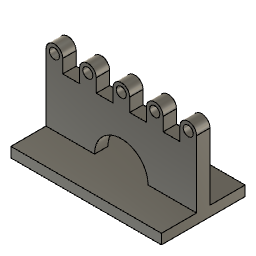
Model 3 (Autodesk Fusion 360 design; units mm, degrees)
Autodesk Fusion 360 part; units mm, degrees
note: some values were not read from the file. Set by a fixed rule: which sketch regions a step uses.
sketch "Sketch5" plane through (0, 0, 0) normal (0, 0, 1) x (1, 0, 0)
  line L0 (0, 0) -> (225, 0)
  line L1 (225, 0) -> (225, -125)
  line L2 (225, -125) -> (0, -125)
  line L3 (0, -125) -> (0, 0)
  dimension "d26" = 225
  dimension "d27" = 125
  constraint horizontal L0
  constraint vertical L1
  constraint horizontal L2
  constraint vertical L3
  constraint coincident L0.start L3.end
  measures "d26" distance of L0.start L0.end
  measures "d27" distance of L0.start L2.end
extrude "Extrude3" add sketch "Sketch5" along normal blind 15
sketch "Sketch6" plane through (0, 0, 15) normal (0, 0, 1) x (-1, 0, 0)
  line L0 (0, 125) -> (-225, 125)
  line L1 (-225, 125) -> (-225, 0)
  line L2 (-225, 0) -> (0, 0)
  line L3 (0, 0) -> (0, 125)
  line L4 (0, 0) -> (0, 62.5) construction
  line L5 (0, 62.5) -> (-225, 62.5) construction
  line L6 (0, 62.5) -> (0, 52.5)
  line L7 (0, 62.5) -> (0, 72.5)
  line L8 (0, 52.5) -> (-225, 52.5)
  line L9 (-225, 52.5) -> (-225, 72.5)
  line L10 (-225, 72.5) -> (0, 72.5)
  dimension "d30" = 62.5
  dimension "d31" = 10
  dimension "d32" = 10
  dimension "d33" = 225
  dimension "d34" = 20
  constraint coincident L2.end L3.start
  constraint perpendicular L0 L4
  constraint midpoint L1 L5.end
  constraint perpendicular L5 L6
  constraint perpendicular L5 L7
  constraint perpendicular L1 L8
  constraint perpendicular L5 L9
  measures "d30" distance of L2.end L4.end
  measures "d31" distance of L4.end L6.end
  measures "d32" distance of L4.end L7.end
  measures "d33" distance of L6.end L8.end
  measures "d34" distance of L8.end L9.end
extrude "Extrude4" add sketch "Sketch6" along normal blind 100 contours L1 L3 L6 L7 L8 L9 L10
sketch "Sketch7" plane through (0, -72.5, 0) normal (0, -1, 0) x (1, 0, 0)
  line L0 (0, 15) -> (225, 15)
  line L1 (225, 15) -> (225, 115)
  line L2 (225, 115) -> (0, 115)
  line L3 (0, 115) -> (0, 15)
  line L4 (0, 15) -> (72.5, 15) construction
  arc A0 (152.5, 15) -> (72.5, 15) centre (112.5, 15) ccw
  line L5 (0, 115) -> (25, 115)
  line L6 (25, 115) -> (50, 115)
  line L7 (50, 115) -> (75, 115)
  line L8 (75, 115) -> (100, 115)
  line L9 (100, 115) -> (125, 115)
  line L10 (125, 115) -> (150, 115)
  line L11 (150, 115) -> (175, 115)
  line L12 (175, 115) -> (200, 115)
  line L13 (200, 115) -> (225, 115)
  circle A1 centre (12.5, 115) radius 7.5
  circle A2 centre (62.5, 115) radius 7.5
  circle A3 centre (112.5, 115) radius 7.5
  circle A4 centre (162.5, 115) radius 7.5
  circle A5 centre (212.5, 115) radius 7.5
  line L14 (25, 115) -> (25, 95)
  line L15 (25, 95) -> (50, 95)
  line L16 (50, 95) -> (50, 115)
  line L17 (75, 115) -> (75, 95)
  line L18 (75, 95) -> (100, 95)
  line L19 (100, 95) -> (100, 115)
  line L20 (125, 115) -> (125, 95)
  line L21 (125, 95) -> (150, 95)
  line L22 (150, 95) -> (150, 115)
  line L23 (175, 115) -> (175, 95)
  line L24 (175, 95) -> (200, 95)
  line L25 (200, 95) -> (200, 115)
  arc A6 (25, 115) -> (0, 115) centre (12.5, 115) ccw
  arc A7 (75, 115) -> (50, 115) centre (62.5, 115) ccw
  arc A8 (125, 115) -> (100, 115) centre (112.5, 115) ccw
  arc A9 (175, 115) -> (150, 115) centre (162.5, 115) ccw
  arc A10 (225, 115) -> (200, 115) centre (212.5, 115) ccw
  point P0 (62.5, 115)
  point P1 (112.5, 115)
  point P2 (162.5, 115)
  point P3 (212.5, 115)
  dimension "d37" = 112.5
  dimension "d38" = 80
  dimension "d42" = 25
  dimension "d43" = 25
  dimension "d44" = 25
  dimension "d45" = 25
  dimension "d46" = 25
  dimension "d47" = 25
  dimension "d48" = 25
  dimension "d49" = 25
  dimension "d50" = 25
  dimension "d51" = 15
  dimension "d52" = 25
  dimension "d55" = 200
  dimension "d56" = 0
  dimension "d57" = 20
  dimension "d62" = 100
  constraint coincident L0.start L3.end
  constraint perpendicular L1 L4
  constraint coincident L0 A0.start
  constraint coincident L2.end L3.start
  constraint perpendicular L3 L5
  constraint parallel L2 L6
  constraint parallel L2 L7
  constraint parallel L2 L8
  constraint parallel L2 L9
  constraint parallel L2 L10
  constraint parallel L2 L11
  constraint parallel L2 L12
  constraint parallel L2 L13
  constraint midpoint L5 A1.centre
  constraint concentric A1 A6
  constraint midpoint L7 P0
  constraint midpoint L9 P1
  constraint midpoint L11 P2
  constraint midpoint L13 P3
  constraint perpendicular L5 L14
  constraint perpendicular L14 L15
  constraint tangent L16 A7
  constraint tangent L17 A7
  constraint perpendicular L8 L17
  constraint perpendicular L17 L18
  constraint tangent L19 A8
  constraint tangent L20 A8
  constraint perpendicular L10 L20
  constraint perpendicular L20 L21
  constraint tangent L22 A9
  constraint tangent L23 A9
  constraint perpendicular L11 L23
  constraint perpendicular L23 L24
  constraint tangent L25 A10
  measures "d37" distance of L0.start A0.centre
  measures "d38" diameter of A0
  measures "d42" distance of L2.end L5.end
  measures "d43" distance of L5.end L6.end
  measures "d44" distance of L6.end L7.end
  measures "d45" distance of L7.end L8.end
  measures "d46" distance of L8.end L9.end
  measures "d47" distance of L9.end L10.end
  measures "d48" distance of L10.end L11.end
  measures "d49" distance of L11.end L12.end
  measures "d50" distance of L12.end L1.end
  measures "d51" diameter of A1
  measures "d52" diameter of A6
  measures "d57" distance of L5.end L14.end
  measures "d62" distance of L0 P3
extrude "Extrude5" cut sketch "Sketch7" against normal blind 20 contours L0 A0
extrude "Extrude6" add sketch "Sketch7" against normal blind 20 contours L2 L5 A1 A6 | L2 L5 A1 | L2 L5 A1 | L2 L7 A2 A7 | L2 L13 A5 A10 | L2 L7 A2 | L2 L13 A5 | L2 L9 A3 A8 | L2 L11 A4 A9 | L2 L9 A3 | L2 L11 A4 picked at (63.3854, 117.6998) picked at (214.3326, 116.7004) picked at (113.3854, 117.6998) picked at (164.3326, 116.7004)
extrude "Extrude7" cut sketch "Sketch7" against normal blind 20 contours L2 L6 L14 L15 L16 | L2 L8 L17 L18 L19 | L2 L12 L23 L24 L25 | L2 L10 L20 L21 L22
extrude "Extrude8" cut sketch "Sketch7" against normal blind 20 contours L2 L5 A1 | L2 L5 A1 | L2 L7 A2 | L2 L7 A2 | L2 L13 A5 | L2 L13 A5 | L2 L9 A3 | L2 L9 A3 | L2 L11 A4 | L2 L11 A4
